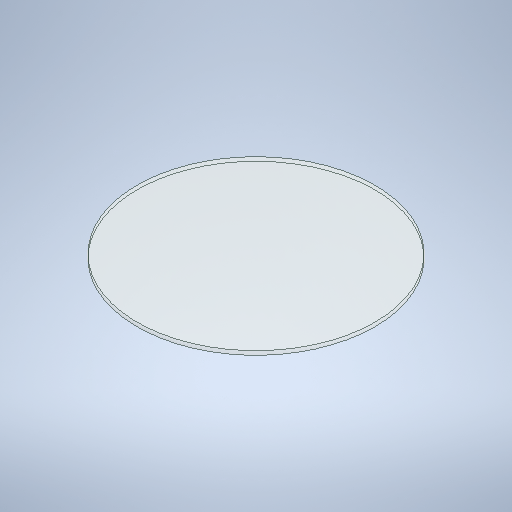
# Autodesk Inventor part: Antireflective Glass
Saved by Autodesk Inventor 2026.2 (Build 302298000, 298)
## iProperties
Created: 2026-03-01
Part Number: Antireflective Glass
Material: Glass
Document SubType Name: Modeling
Designer: mumin
Density: 2.18 g/cm^3
Appearance: Clear
Author: mumin
Autodesk Inventor part; units mm, degrees
ref_plane "YZ Plane" through (0, 0, 0) normal (1, 0, 0) x (0, 1, 0)
ref_plane "XZ Plane" through (0, 0, 0) normal (0, 1, 0) x (-1, 0, 0)
ref_plane "XY Plane" through (0, 0, 0) normal (0, 0, 1) x (1, 0, 0)
sketch "Sketch2" plane through (0, 0, 0) normal (0, 0, 1) x (1, 0, 0)
  line L0 (0, 0) -> (0, 37.9803)
  line L1 (0, 2) -> (119.2553, 2)
  line L2 (119.2553, 2) -> (119.2553, -2)
  line L3 (119.2553, -2) -> (0, -2)
  line L4 (0, -2) -> (0, 2)
  line L5 (-24, 0) -> (144, 0) projected
  arc A0 (119.2553, -2) -> (119.2553, 2) centre (116.942, 0) ccw
  line L6 (120, 0) -> (120, 4.9863) construction
  point P0 (119.2553, 0)
  dimension "d3" = 4
  dimension "d4" = 240
  constraints: 12 end point, 3 point on circle, 2 parallel, 2 point on line, 2 vertical, 1 centre point, 1 horizontal, 1 midpoint, 1 perpendicular, 1 tangent
  measures "d3" distance of L1.end L2.end
  measures "d4" diameter of L6 L0
revolve "Revolution1" add sketch "Sketch2" angle 360 about axis through (0, 0, 0) along (0, 1, 0)
body "Solid2"
